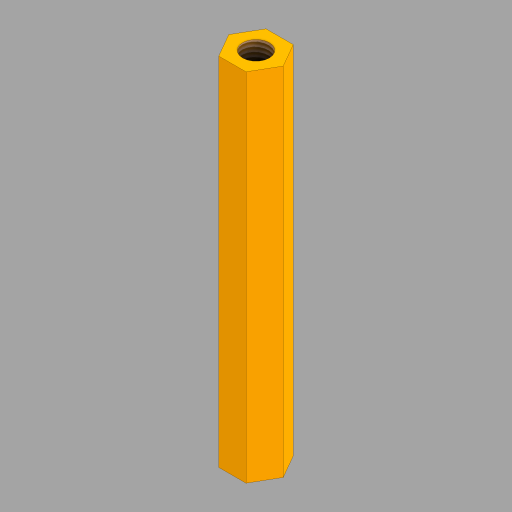
# Autodesk Inventor part: stoyka_30mm
Saved by Autodesk Inventor 2024.2 (Build 282272000, 272)
## iProperties
Created: 2023-12-16
Part Number: stoyka_30mm
Material: Типовые
Document SubType Name: Modeling
Designer: Фёдор
Density: 1 g/cm^3
Appearance: По умолчанию
Author: Фёдор
Autodesk Inventor part; units mm, degrees
ref_plane "YZ Plane" through (0, 0, 0) normal (1, 0, 0) x (0, 1, 0)
ref_plane "XZ Plane" through (0, 0, 0) normal (0, 1, 0) x (-1, 0, 0)
ref_plane "XY Plane" through (0, 0, 0) normal (0, 0, 1) x (1, 0, 0)
sketch "Эскиз1" plane through (0, 0, 0) normal (0, 1, 0) x (-1, 0, 0)
  circle A0 centre (0, 0) radius 1.5
  line L0 (3.06, 0) -> (1.53, -2.65)
  line L1 (1.53, -2.65) -> (-1.53, -2.65)
  line L2 (-1.53, -2.65) -> (-3.06, 0)
  line L3 (-3.06, 0) -> (-1.53, 2.65)
  line L4 (-1.53, 2.65) -> (1.53, 2.65)
  line L5 (1.53, 2.65) -> (3.06, 0)
  dimension "d0" = 3
  dimension "d1" = 5.3
  dimension "d2" = 5.3
  constraints: 12 end point, 2 coincident, 1 centre point, 13 other
  measures "d0" diameter of A0
  measures "d1" distance between parallel lines of L0 L3
  measures "d2" vertical distance of L0.end L3.end
extrude "Выдавливание1" add sketch "Эскиз1" along normal blind 40
thread "Резьба1" size "M3x0.5" class "6H" standard "ANSI Metric M Profile" full length
equation "\"d1\" = d2"
